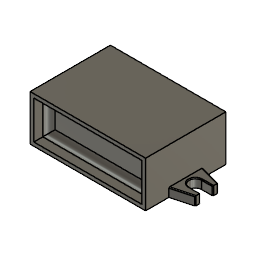
mirror (Autodesk Fusion 360 archive; units mm, degrees)
design "DC-DC Converter"
Autodesk Fusion 360 part; units mm, degrees
sketch "Sketch1" plane through (0, 0, 0) normal (0, 0, 1) x (1, 0, 0)
  line L0 (0, 0) -> (46, 0)
  line L1 (46, 0) -> (46, -32)
  line L2 (46, -32) -> (0, -32)
  line L3 (0, -32) -> (0, 0)
  dimension "d1" = 46
  dimension "d2" = 32
  constraint coincident L0.start L3.end
  constraint horizontal L0
  constraint perpendicular L0 L1
  constraint perpendicular L1 L2
  constraint perpendicular L0 L3
  measures "d1" distance of L0.start L0.end
  measures "d2" distance of L0.end L1.end
extrude "Extrude1" add sketch "Sketch1" along normal blind 18.16
sketch "Sketch2" plane through (0, 0, 0) normal (0, 0, -1) x (1, 0, 0)
  line L0 (46, 32) -> (0, 32)
  line L1 (0, 32) -> (0, 0)
  line L2 (0, 0) -> (46, 0)
  line L3 (46, 0) -> (46, 32)
  line L4 (23, 0) -> (23, 32)
  line L5 (23, 16) -> (-1.31, 16)
  line L6 (23, 16) -> (47.31, 16)
  line L7 (47.31, 16) -> (54.31, 16)
  circle A0 centre (49.81, 16) radius 2.5
  line L8 (-1.31, 16) -> (-8.31, 16)
  circle A1 centre (-3.81, 16) radius 2.5
  line L9 (-8.31, 16) -> (-8.31, 13.5)
  line L10 (-8.31, 16) -> (-8.31, 18.5)
  line L11 (-3.81, 16) -> (-3.81, 18.5)
  line L12 (-3.81, 18.5) -> (-8.31, 18.5)
  line L13 (-3.81, 16) -> (-3.81, 13.5)
  line L14 (-3.81, 13.5) -> (-8.31, 13.5)
  line L15 (49.81, 16) -> (49.81, 18.5)
  line L16 (49.81, 16) -> (49.81, 13.5)
  line L17 (54.31, 16) -> (54.31, 13.5)
  line L18 (49.81, 13.5) -> (54.31, 13.5)
  line L19 (54.31, 16) -> (54.31, 18.5)
  line L20 (49.81, 18.5) -> (54.31, 18.5)
  line L21 (56.31, 16) -> (56.31, 20.5)
  line L22 (47.81, 20.5) -> (56.31, 20.5)
  line L23 (47.81, 16) -> (47.81, 20.5)
  line L24 (47.81, 16) -> (47.81, 11.5)
  line L25 (47.81, 11.5) -> (56.31, 11.5)
  line L26 (56.31, 16) -> (56.31, 11.5)
  line L27 (54.31, 13.5) -> (54.31, 11.5)
  line L28 (-1.81, 16) -> (-1.81, 11.5)
  line L29 (-1.81, 11.5) -> (-10.31, 11.5)
  line L30 (-10.31, 16) -> (-10.31, 11.5)
  line L31 (-10.31, 16) -> (-10.31, 20.5)
  line L32 (-1.81, 20.5) -> (-10.31, 20.5)
  line L33 (-1.81, 16) -> (-1.81, 20.5)
  line L34 (-8.31, 13.5) -> (-8.31, 11.5)
  line L35 (-8.31, 18.5) -> (-8.31, 20.5)
  line L36 (-8.31, 20.5) -> (0, 22.7267)
  line L37 (-8.31, 20.5) -> (0.2931, 20.5) construction
  line L38 (-8.31, 11.5) -> (0, 9.2733)
  line L39 (-8.31, 11.5) -> (0.2931, 11.5) construction
  line L40 (54.31, 11.5) -> (46, 9.2733)
  line L41 (54.31, 11.5) -> (62.9131, 11.5) construction
  line L42 (54.31, 20.5) -> (46, 22.7267)
  line L43 (54.31, 20.5) -> (62.9131, 20.5) construction
  line L44 (54.31, 20.5) -> (54.31, 18.5)
  dimension "d5" = 24.31
  dimension "d6" = 24.31
  dimension "d7" = 7
  dimension "d8" = 5
  dimension "d9" = 7
  dimension "d10" = 5
  dimension "d11" = -2
  dimension "d12" = -2
  dimension "d13" = 15
  dimension "d14" = 15
  dimension "d15" = 165
  dimension "d16" = 165
  constraint midpoint L2 L4.start
  constraint perpendicular L2 L4
  constraint midpoint L4 L5.start
  constraint perpendicular L4 L5
  constraint perpendicular L4 L6
  constraint perpendicular L3 L7
  constraint coincident L6.end A0
  constraint horizontal L8
  constraint coincident L5.end A1
  constraint perpendicular L8 L9
  constraint perpendicular L8 L10
  constraint coincident A1.centre L11.start
  constraint coincident A1 L11.end
  constraint perpendicular L8 L11
  constraint tangent A1 L12
  constraint coincident A1 L13.end
  constraint perpendicular L8 L13
  constraint coincident A0.centre L15.start
  constraint coincident A0 L15.end
  constraint perpendicular L7 L15
  constraint coincident A0 L16.end
  constraint perpendicular L7 L16
  constraint perpendicular L7 L17
  constraint tangent A0 L18
  constraint perpendicular L7 L19
  constraint coincident L25 L27.end
  constraint perpendicular L25 L27
  constraint coincident L29 L34.end
  constraint perpendicular L29 L34
  constraint coincident L32 L35.end
  constraint perpendicular L32 L35
  constraint horizontal L37
  constraint coincident L1 L36.end
  constraint horizontal L39
  constraint coincident L1 L38.end
  constraint horizontal L41
  constraint coincident L3 L40.end
  constraint horizontal L43
  constraint coincident L22 L42.start
  constraint coincident L3 L42.end
  constraint parallel L19 L44
  measures "d5" distance of L5.start L5.end
  measures "d6" distance of L5.start L6.end
  measures "d7" distance of L6.end L7.end
  measures "d8" diameter of A0
  measures "d9" distance of L5.end L8.end
  measures "d10" diameter of A1
  measures "d13" angle of L36 L37
  measures "d14" angle of L38 L39
  measures "d15" angle of L40 L41
  measures "d16" angle of L42 L43
extrude "Extrude2" add sketch "Sketch2" against normal blind 3.5 contours L3 L6 A0 L22 L23 L42 | L3 L6 A0 L24 L25 L40 | A0 L20 L22 L23 L44 | L1 L5 A1 L32 L33 L36 | L1 L5 A1 L28 L29 L38 | A1 L12 L32 L33 L35 | A0 L18 L24 L25 L27 | A1 L14 L28 L29 L34
fillet "Fillet1" radius 0.3 18 edges at (-8.31, -11.5, 1.75) (-8.31, -13.5, 1.75) (-8.31, -18.5, 1.75) (-8.31, -20.5, 1.75) (-6.06, -13.5, 3.5) (-1.31, -16, 3.5) (-6.06, -18.5, 3.5) (-4.155, -10.3867, 3.5) (-4.155, -21.6133, 3.5) (50.155, -10.3867, 3.5) (52.06, -18.5, 3.5) (47.31, -16, 3.5) (52.06, -13.5, 3.5) (54.31, -13.5, 1.75) (54.31, -11.5, 1.75) (54.31, -18.5, 1.75) (54.31, -20.5, 1.75) (50.155, -21.6133, 3.5)
sketch "Sketch3" plane through (0, -32, 0) normal (0, -1, 0) x (1, 0, 0)
  line L0 (0, 0) -> (46, 0)
  line L1 (46, 0) -> (46, 18.16)
  line L2 (46, 18.16) -> (0, 18.16)
  line L3 (0, 18.16) -> (0, 0)
  line L4 (1.5, 1.5) -> (44.5, 1.5)
  line L5 (44.5, 1.5) -> (44.5, 16.66)
  line L6 (44.5, 16.66) -> (1.5, 16.66)
  line L7 (1.5, 16.66) -> (1.5, 1.5)
  dimension "d21" = -1.5
extrude "Extrude3" cut sketch "Sketch3" against normal blind 4.369 contours L4 L5 L6 L7
extrude "Extrude4" cut 1 faces at (15.8333, -27.631, 11.6067) along direction (0, 1, 0) blind 1.648
fillet "Fillet2" radius 2.458 4 edges at (23, -25.983, 1.5) (44.5, -25.983, 9.08) (23, -25.983, 16.66) (1.5, -25.983, 9.08)
equation "d5 = ( 48.62 / 2 ) * 1 mm"
equation "d6 = ( 48.62 / 2 ) * 1 mm"

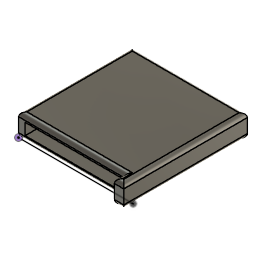
design "computer"
Autodesk Fusion 360 part; units mm, degrees
sketch "Sketch1" plane through (0, 0, 0) normal (0, 0, 1) x (1, 0, 0)
  line L0 (0, 0) -> (176.2125, 0)
  dimension "d1" = 176.2125
  constraint coincident L0.start origin
  constraint horizontal L0
  measures "d1" distance of L0.start L0.end
sketch "Sketch2" plane through (0, 0, 0) normal (0, 0, 1) x (1, 0, 0)
  line L0 (0, 0) -> (177.038, 0)
  line L1 (177.038, 0) -> (177.038, 174.752)
  line L2 (0, 0) -> (177.038, 0)
  line L3 (177.038, 0) -> (177.038, 174.752)
  line L4 (177.038, 174.752) -> (0, 174.752)
  line L5 (0, 174.752) -> (0, 0)
  dimension "d2" = 177.038
  dimension "d3" = 174.752
  constraint coincident L0.start L2.start
  constraint horizontal L0
  constraint perpendicular L0 L1
  constraint horizontal L2
  constraint vertical L3
  constraint horizontal L4
  constraint vertical L5
  measures "d2" distance of L0.start L0.end
  measures "d3" distance of L0.end L1.end
extrude "Extrude1" add sketch "Sketch2" along normal blind 34.29
sketch "Sketch3" plane through (0, 0, 0) normal (0, -1, 0) x (1, 0, 0)
  line L0 (0, 0) -> (177.038, 0)
  line L1 (177.038, 0) -> (177.038, 34.29)
  line L2 (177.038, 34.29) -> (0, 34.29)
  line L3 (0, 34.29) -> (0, 0)
  line L4 (165.1, 7.62) -> (10.16, 7.62)
  line L5 (10.16, 7.62) -> (10.16, 25.4)
  line L6 (10.16, 25.4) -> (165.1, 25.4)
  line L7 (165.1, 25.4) -> (165.1, 7.62)
  constraint horizontal L4
  constraint vertical L5
  constraint horizontal L6
  constraint vertical L7
extrude "Extrude2" cut sketch "Sketch3" against normal blind 24.7142 contours L4 L5 L6 L7
sketch "Sketch4" plane through (0, 0, 0) normal (0, 0, -1) x (1, 0, 0)
  line L0 (0, 0) -> (0, -174.752)
  line L1 (0, -174.752) -> (177.038, -174.752)
  line L2 (177.038, -174.752) -> (177.038, 0)
  line L3 (177.038, 0) -> (0, 0)
  line L4 (177.038, 0) -> (162.56, 0)
  line L5 (162.56, 0) -> (162.56, 15.24)
  line L6 (162.56, 15.24) -> (177.038, 15.24)
  line L7 (177.038, 15.24) -> (177.038, 0)
  constraint horizontal L4
  constraint vertical L5
  constraint horizontal L6
  constraint vertical L7
  constraint coincident L2.end L3.start
extrude "Extrude3" add sketch "Sketch4" against normal blind 34.29 contours L3 L4 L5 L6 L7
fillet "Fillet1" radius 6.477 12 edges at (81.28, 0, 0) (0, 87.376, 0) (0, 87.376, 34.29) (81.28, 0, 34.29) (162.56, -7.62, 34.29) (169.799, -15.24, 34.29) (169.799, -15.24, 0) (162.56, -7.62, 0) (177.038, 79.756, 0) (177.038, 79.756, 34.29) (88.519, 174.752, 34.29) (88.519, 174.752, 0)
equation "d1 = 7 in - ( ( 1 / 16 ) * 1 in )"
